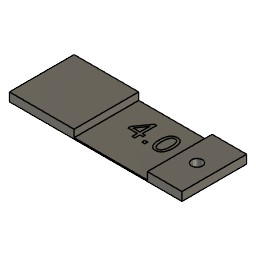
Thickness-4.0 mm (Autodesk Fusion 360 design; units mm, degrees)
Autodesk Fusion 360 part; units mm, degrees
sketch "Schizzo1" plane through (0, 0, 0) normal (0, 0, 1) x (1, 0, 0)
  line L0 (-35.7529, 16.0578) -> (-5.7529, 16.0578)
  line L1 (-5.7529, 16.0578) -> (-5.7529, -13.9422)
  line L2 (-5.7529, -13.9422) -> (-35.7529, -13.9422)
  line L3 (-35.7529, -13.9422) -> (-35.7529, 16.0578)
  line L4 (-5.7529, 16.0578) -> (44.2471, 16.0578)
  line L5 (44.2471, 16.0578) -> (44.2471, -13.9422)
  line L6 (44.2471, -13.9422) -> (-5.7529, -13.9422)
  line L7 (36.2471, 16.0578) -> (36.2471, -13.9422) construction
  line L8 (44.2471, 1.0578) -> (-5.7529, 1.0578) construction
  circle A0 centre (36.2471, 1.0578) radius 2.5
  line L9 (28.2471, 16.0578) -> (28.2471, -13.9422)
  line L10 (6.9284, 1.1522) -> (17.2791, 1.0578) construction
  line L11 (17.2791, 1.0578) -> (17.3507, 8.9056) construction
  line L12 (17.3507, 8.9056) -> (7, 9) construction
  line L13 (7, 9) -> (6.9284, 1.1522) construction
  dimension "d1" = 30
  dimension "d2" = 30
  dimension "d3" = 50
  dimension "d4" = 30
  dimension "d5" = 8
  dimension "d6" = 5
  dimension "d13" = 8
  dimension "d14" = 10
  dimension "d15" = 0
  text T0 "4.0" font "Arial" height 10 align centre middle in box 10.3512 x 7.8481 at (6.9284, 1.1522) x (0.999958, -0.009124) y (0.009124, 0.999958) spacing 1 kerned
  constraint horizontal L0
  constraint vertical L1
  constraint horizontal L2
  constraint vertical L3
  constraint perpendicular L1 L4
  constraint perpendicular L4 L5
  constraint coincident L4 L7.start
  constraint coincident L6 L7.end
  constraint perpendicular L6 L7
  constraint midpoint L5 L8.start
  constraint midpoint L1 L8.end
  constraint midpoint L7 A0.centre
  constraint coincident L4 L9.start
  constraint coincident L6 L9.end
  constraint perpendicular L6 L9
  constraint coincident L8
  measures "d1" distance of L0.start L0.end
  measures "d2" distance of L0.start L2.end
  measures "d3" distance of L0.end L4.end
  measures "d4" distance of L4.end L5.end
  measures "d5" distance of L5 L7
  measures "d6" diameter of A0
  measures "d13" distance of L7 L9
extrude "Estrusione1" add sketch "Schizzo1" along normal blind 4 contours L0 L1 L2 L3 makes body 1
extrude "Estrusione2" add sketch "Schizzo1" along normal blind 0.6 contours L1 L4 L6 L9 bodies 1
extrude "Estrusione3" add sketch "Schizzo1" along normal up to surface (4 mm away) contours L4 L5 L6 L9 bodies 1
extrude "Estrusione4" add sketch "Schizzo1" along normal up to surface (0.6 mm away) separate body text T0 makes body 2 at (15.7655, 4.0516, 0) makes body 3 at (12.6041, 0.4906, 0) makes body 4 at (8.0294, 7.2493, 0)
extrude "Estrusione5" cut sketch "Schizzo1" along normal blind 5.5 text T0 bodies 1 makes body 5 at (6.1475, 5.1063, 0.6) makes body 6 at (-22.8923, 1.5412, 0)
equation "d13 = d5"
equation "d15 = '4.0'"
